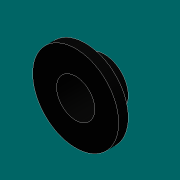
# Autodesk Inventor part: D4050-9120B
Saved by Autodesk Inventor 2016 (Build 200138000, 138)
## iProperties
Created: 2016-08-26
Part Number: D4050-9120B
Material: アセタール樹脂、黒
Document SubType Name: Modeling
Designer: hiro
Density: 1.425 g/cm^3
Appearance: 滑らか - 黒
Mass: 0.092893 g
Surface Area: 1.99491 cm^2
Volume: 0.065188 cm^3
Author: hiro
Autodesk Inventor part; units mm, degrees
ref_plane "YZ Plane" through (0, 0, 0) normal (1, 0, 0) x (0, 1, 0)
ref_plane "XZ Plane" through (0, 0, 0) normal (0, 1, 0) x (-1, 0, 0)
ref_plane "XY Plane" through (0, 0, 0) normal (0, 0, 1) x (1, 0, 0)
sketch "スケッチ1" plane through (0, 0, 0) normal (0, 0, 1) x (1, 0, 0)
  line L0 (2, 1.5) -> (2, -1.5)
  line L1 (2, -1.5) -> (4.5, -1.5)
  line L2 (4.5, -1.5) -> (4.5, -0.5)
  line L3 (4.5, -0.5) -> (2.5, -0.5)
  line L4 (2.5, -0.5) -> (2.5, 1.5)
  line L5 (2.5, 1.5) -> (2, 1.5)
  line L6 (0, 1.5) -> (0, -1.5) construction
  point P0 (0, 0)
  point P1 (0, 0)
  point P2 (2, 0)
  dimension "d0" = 4
  dimension "d1" = 5
  dimension "d2" = 1
  dimension "d3" = 2
  dimension "d4" = 9
  constraints: 14 end point, 5 perpendicular, 2 midpoint, 2 vertical, 1 coincident, 1 horizontal alignment, 1 point on line
  measures "d0" diameter of L0 L6
  measures "d1" diameter of L4 L6
  measures "d2" distance of L1.end L2.end
  measures "d3" distance of L3.end L4.end
  measures "d4" diameter of L2 L6
revolve "回転1" add sketch "スケッチ1" angle 360 about axis through (0, 1.5, 0) along (0, -1, 0)
